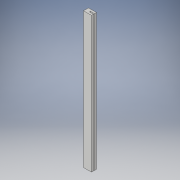
# Autodesk Inventor part: window frame short
Saved by Autodesk Inventor 2017 (Build 210142000, 142)
## iProperties
Created: 2019-05-07
Part Number: window frame short
Material: Generic
Document SubType Name: Modeling
Designer: Roman
Density: 1 g/cm^3
Appearance: Default
Author: Roman
Autodesk Inventor part; units mm, degrees
ref_plane "YZ Plane" through (0, 0, 0) normal (1, 0, 0) x (0, 1, 0)
ref_plane "XZ Plane" through (0, 0, 0) normal (0, 1, 0) x (-1, 0, 0)
ref_plane "XY Plane" through (0, 0, 0) normal (0, 0, 1) x (1, 0, 0)
sketch "Sketch1" plane through (0, 0, 0) normal (0, 1, 0) x (-1, 0, 0)
  line L0 (0, 0) -> (-25.4, 0)
  line L1 (-25.4, 0) -> (-25.4, -6.35)
  line L2 (-25.4, -6.35) -> (0, -6.35)
  line L3 (0, -6.35) -> (0, 0)
  line L4 (0, -6.35) -> (-12.7, -6.35)
  line L5 (-12.7, -6.35) -> (-12.7, -9.525)
  line L6 (-12.7, -9.525) -> (0, -9.525)
  line L7 (0, -9.525) -> (0, -6.35)
  line L8 (0, -9.525) -> (-25.4, -9.525)
  line L9 (-25.4, -9.525) -> (-25.4, -15.875)
  line L10 (-25.4, -15.875) -> (0, -15.875)
  line L11 (0, -15.875) -> (0, -9.525)
  dimension "d0" = 25.4
  dimension "d1" = 6.35
  dimension "d2" = 12.7
  dimension "d3" = 3.175
  dimension "d4" = 25.4
  dimension "d5" = 6.35
  constraints: 24 end point, 6 parallel, 3 horizontal, 3 perpendicular
  measures "d0" distance of L2.end L1.end
  measures "d1" distance of L1.end L0.end
  measures "d2" distance of L6.end L5.end
  measures "d3" distance of L5.end L4.end
  measures "d4" distance of L10.end L9.end
  measures "d5" distance of L9.end L8.end
extrude "Extrusion1" add sketch "Sketch1" along normal blind 431.8
body "Solid1"
